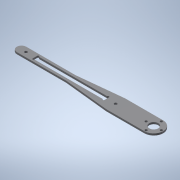
# Autodesk Inventor part: ForeArm_outside_frame
Saved by Autodesk Inventor 2020.4 (Build 244396000, 396)
## iProperties
Created: 2016-05-04
Part Number: ForeArm_outside_frame
Material: GFRP
Document SubType Name: Modeling
Designer: hiroaki
Density: 1.75 g/cm^3
Appearance: 滑らか - 淡い灰色
Mass: 10.0158 g
Surface Area: 72.6648 cm^2
Volume: 5.7233 cm^3
Description: GFRP T2
d0: 147.500 mm
d1: 3.100 mm
d2: 21.000 mm
d3: 10.000 mm
d4: 5.000 mm
d5: 12.000 mm
d6: 100.000 mm
d7: 5.000 mm
d8: 0.050 mm
d9: 2.100 mm
d10: 2.700 mm
d11: 8.500 mm
d12: 10.100 mm
d13: 4.000 ul
d15: 360.00 deg
d17: 2.000 mm
d18: 0.00 deg
d19: 2.000 mm
Author: hiroaki
Autodesk Inventor part; units mm, degrees
ref_plane "YZ Plane" through (0, 0, 0) normal (1, 0, 0) x (0, 1, 0)
ref_plane "XZ Plane" through (0, 0, 0) normal (0, 1, 0) x (-1, 0, 0)
ref_plane "XY Plane" through (0, 0, 0) normal (0, 0, 1) x (1, 0, 0)
sketch "スケッチ1" plane through (0, 0, 0) normal (0, 0, 1) x (1, 0, 0)
  circle A0 centre (0, 0) radius 10.5 construction
  line L0 (0, 10.5) -> (-147.5, 10.5) construction
  line L1 (-147.5, 10.5) -> (-147.5, -10.5) construction
  line L2 (-147.5, -10.5) -> (0, -10.5) construction
  circle A1 centre (-142.5, 0) radius 1.55
  line L3 (-132.5, 2.5) -> (-52.5, 2.5) construction
  line L4 (-52.5, 2.5) -> (-52.5, -2.5) construction
  line L5 (-52.5, -2.5) -> (-132.5, -2.5) construction
  line L6 (-132.5, -2.5) -> (-132.5, 2.5) construction
  line L7 (-92.5, 2.5) -> (-92.5, -2.5) construction
  circle A2 centre (-42.5, 0) radius 1.55
  line L8 (-12, 21.3027) -> (-12, -27.3903) construction
  line L9 (-52.45, 2.55) -> (-132.55, 2.55) construction
  line L10 (-132.55, 2.55) -> (-132.55, -2.55) construction
  line L11 (-132.55, -2.55) -> (-52.45, -2.55) construction
  line L12 (-52.45, -2.55) -> (-52.45, 2.55) construction
  circle A3 centre (-131.5, 2.55) radius 1.05 construction
  line L13 (-132.5, 0) -> (-92.5, 0) construction
  line L14 (-132.55, 2.55) -> (-132.55, -2.55)
  arc A4 (-130.45, 2.55) -> (-132.55, 2.55) centre (-131.5, 2.55) ccw
  line L15 (-130.45, 2.55) -> (-54.55, 2.55)
  arc A5 (-52.45, 2.55) -> (-54.55, 2.55) centre (-53.5, 2.55) ccw
  line L16 (-52.45, 2.55) -> (-52.45, -2.55)
  arc A6 (-132.55, -2.55) -> (-130.45, -2.55) centre (-131.5, -2.55) ccw
  line L17 (-130.45, -2.55) -> (-54.55, -2.55)
  arc A7 (-54.55, -2.55) -> (-52.45, -2.55) centre (-53.5, -2.55) ccw
  circle A8 centre (0, 8.5) radius 1.35
  circle A9 centre (0, 0) radius 5.05
  circle A10 centre (-8.5, 0) radius 1.35
  circle A11 centre (0, -8.5) radius 1.35
  circle A12 centre (8.5, 0) radius 1.35
  line L18 (-42.5, 10.5) -> (0, 10.5)
  line L19 (-42.5, -10.5) -> (0, -10.5)
  arc A13 (0, -10.5) -> (0, 10.5) centre (0, 0) ccw
  circle A14 centre (-142.5, 0) radius 5 construction
  arc A15 (-147.5, 5.25) -> (-147.5, -5.25) centre (-147.5, 0) ccw
  line L20 (-147.5, 5.25) -> (-92.5, 5.25)
  line L21 (-92.5, 5.25) -> (-42.5, 10.5)
  line L22 (-147.5, -5.25) -> (-92.5, -5.25)
  line L23 (-92.5, -5.25) -> (-42.5, -10.5)
  dimension "d9" = 2.1
  dimension "d0" = 147.5
  dimension "d1" = 3.1
  dimension "d2" = 21
  dimension "d3" = 10
  dimension "d4" = 5
  dimension "d5" = 12
  dimension "d6" = 100
  dimension "d7" = 5
  dimension "d8" = 0.05
  dimension "d10" = 2.7
  dimension "d11" = 8.5
  dimension "d12" = 10.1
  dimension "d15" = 360
  dimension "d20" = 5.25
  dimension "d21" = 50
  constraints: 48 end point, 14 centre point, 14 point on circle, 7 tangent, 6 coincident, 6 horizontal, 6 symmetric about line, 5 midpoint, 4 horizontal alignment, 4 parallel, 4 perpendicular, 3 equal radius, 3 point on line, 3 vertical, 2 vertical alignment, 1 collinear, 1 concentric, 18 other
  measures "d0" distance from line of L1 point (0, 0)
  measures "d1" diameter of A1
  measures "d2" distance of L0.end L1.end
  measures "d3" distance from line of L6 A1.centre
  measures "d4" distance from line of L1 A1.centre
  measures "d5" distance from line of point (0, 0) L8
  measures "d6" distance of A2.centre A1.centre
  measures "d7" distance of L3.end L4.end
  measures "d8" distance between parallel lines of L9 L3
  measures "d10" diameter of A8
  measures "d11" distance of point (0, 0) A8.centre
  measures "d12" diameter of A9
  measures "d20" distance from line of L22 A1.centre
  measures "d21" horizontal distance of L20.end A1.centre
extrude "押し出し1" add sketch "スケッチ1" along normal blind 2
fillet "フィレット1" radius 2 2 edges at (-92.5, -5.25, 1) (-92.5, 5.25, 1)
equation "\"H_head\" = 28.5"
equation "\"H_leg\" = 199.5"
equation "\"足の面積\" = 12720.125"
equation "\"現在の面積\" = 11560"
equation "\"足_短辺\" = 68"
equation "\"円柱\" = 313.5"
equation "\"胴体中心から手先\" = 342"
equation "\"H_leg_1\" = 186.2"
equation "\"H_leg_MAX\" = 399"
equation "\"H_head_1\" = 26.6"
equation "\"H_head_MAX\" = 142.5"
